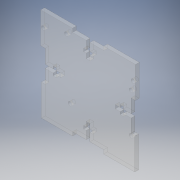
# Autodesk Inventor part: pared lateral
Saved by Autodesk Inventor 2016 (Build 200138000, 138)
## iProperties
Created: 2017-02-20
Part Number: pared lateral
Material: Generic
Document SubType Name: Modeling
Designer: jorge
Density: 1 g/cm^3
Appearance: Clear - Light
Author: jorge
## iProperties of the stored document pared lateral_3DPrint.ipt
Created: 2017-03-11
Part Number: pared lateral_3DPrint
Material: Generic
Document SubType Name: Modeling
Designer: jorge
Density: 1 g/cm^3
Appearance: Default
Author: jorge
Autodesk Inventor part; units mm, degrees
ref_plane "YZ Plane" through (0, 0, 0) normal (1, 0, 0) x (0, 1, 0)
ref_plane "XZ Plane" through (0, 0, 0) normal (0, 1, 0) x (-1, 0, 0)
ref_plane "XY Plane" through (0, 0, 0) normal (0, 0, 1) x (1, 0, 0)
sketch "Sketch1" plane through (0, 0, 0) normal (0, 0, 1) x (1, 0, 0)
  line L0 (0, 0) -> (25, 0) projected
  line L1 (25, 0) -> (25, 3) projected
  line L2 (0, 3) -> (25, 3) projected
  line L3 (0, 0) -> (0, 3) projected
  line L4 (25, 0) -> (50, 0) projected
  line L5 (50, 0) -> (50, 3) projected
  line L6 (25, 3) -> (50, 3) projected
  line L7 (25, 0) -> (25, 3) projected
  line L8 (50, 0) -> (75, 0) projected
  line L9 (75, 0) -> (75, 3) projected
  line L10 (50, 3) -> (75, 3) projected
  line L11 (50, 0) -> (50, 3) projected
  line L12 (0, 0) -> (0, 75)
  line L13 (0, 75) -> (75, 75)
  line L14 (75, 75) -> (75, 0)
  line L15 (75, 0) -> (50, 0)
  line L16 (50, 3) -> (50, 0)
  line L17 (50, 3) -> (25, 3)
  line L18 (25, 3) -> (25, 0)
  line L19 (25, 0) -> (0, 0)
  line L20 (0, 0) -> (0, 25)
  line L21 (0, 25) -> (3, 25)
  line L22 (3, 25) -> (3, 50)
  line L23 (3, 50) -> (0, 50)
  line L24 (25, 75) -> (25, 72)
  line L25 (25, 72) -> (50, 72)
  line L26 (50, 75) -> (50, 72)
  line L27 (75, 50) -> (72, 50)
  line L28 (72, 50) -> (72, 25)
  line L29 (72, 25) -> (75, 25)
  dimension "d0" = 75
  dimension "d1" = 75
  dimension "d2" = 25
  dimension "d3" = 3
  dimension "d4" = 25
  dimension "d5" = 3
  dimension "d6" = 3
  constraints: 36 end point, 11 perpendicular, 6 point on line, 2 collinear, 2 vertical, 1 horizontal
  measures "d0" distance of L0.start L12.end
  measures "d1" distance of L12.end L13.end
  measures "d2" distance of L0.start L20.end
  measures "d3" distance of L20.end L21.end
  measures "d4" distance of L21.end L22.end
  measures "d5" distance of L24.start L24.end
  measures "d6" distance of L27.start L27.end
extrude "Extrusion1" add sketch "Sketch1" along normal blind 3 contours L3 L2 L1 L0 | L12 L21 L22 L23 L13 L24 L25 L26 L14 L27 L28 L29 L10 L6 L2 | L5 L10 L9 L8
sketch "Sketch2" plane through (0, 0, 0) normal (0, 0, -1) x (-1, 0, 0)
  circle A0 centre (-72, 55.2929) radius 1.5 projected
  circle A1 centre (-20, 68.5) radius 1.5 projected
  circle A2 centre (-23, 21.5) radius 1.5 projected
  circle A3 centre (-72, 23.7071) radius 1.5 projected
  point P0 (0, 0)
extrude "Extrusion2" cut sketch "Sketch2" against normal blind 25.4
sketch "Sketch3" plane through (0, 0, 0) normal (0, 0, -1) x (-1, 0, 0)
  line L0 (-50, 72) -> (-39, 72) projected
  line L1 (-25, 72) -> (-25, 75) projected
  line L2 (-25, 75) -> (0, 75) projected
  line L3 (0, 62.5) -> (0, 50) projected
  line L4 (0, 50) -> (-3, 50) projected
  line L5 (-3, 50) -> (-3, 39) projected
  line L6 (-3, 25) -> (0, 25) projected
  line L7 (0, 25) -> (0, 0) projected
  line L8 (0, 0) -> (-25, 0) projected
  line L9 (-25, 0) -> (-25, 3) projected
  line L10 (-25, 3) -> (-36, 3) projected
  line L11 (-50, 3) -> (-50, 0) projected
  line L12 (-50, 0) -> (-75, 0) projected
  line L13 (-75, 0) -> (-75, 25) projected
  line L14 (-75, 25) -> (-72, 25) projected
  line L15 (-72, 25) -> (-72, 36) projected
  line L16 (-72, 50) -> (-75, 50) projected
  line L17 (-75, 62.5) -> (-75, 75) projected
  line L18 (-75, 75) -> (-50, 75) projected
  line L19 (-50, 75) -> (-50, 72) projected
  circle A0 centre (-19, 19.65) radius 1.5 projected
  circle A1 centre (-19, 56.95) radius 1.5 projected
  circle A2 centre (-56.3, 56.95) radius 1.5 projected
  circle A3 centre (-56.3, 19.65) radius 1.5 projected
  line L20 (-39, 72) -> (-36, 72)
  line L21 (-3, 39) -> (-3, 36)
  line L22 (-3, 50) -> (-3, 25) projected
  line L23 (-39, 3) -> (-36, 3)
  line L24 (-25, 3) -> (-50, 3) projected
  line L25 (-72, 36) -> (-72, 39)
  line L26 (-72, 25.2071) -> (-72, 50) projected
  line L27 (-72, 39) -> (-72, 50) projected
  line L28 (-36, 72) -> (-25, 72) projected
  line L29 (-3, 36) -> (-3, 25) projected
  line L30 (-39, 3) -> (-50, 3) projected
  line L31 (-72, 36) -> (-65.65, 36) projected
  line L32 (-65.65, 36) -> (-65.65, 34) projected
  line L33 (-65.65, 34) -> (-63.15, 34) projected
  line L34 (-63.15, 34) -> (-63.15, 36) projected
  line L35 (-63.15, 36) -> (-59.3, 36) projected
  line L36 (-59.3, 36) -> (-59.3, 39) projected
  line L37 (-59.3, 39) -> (-63.15, 39) projected
  line L38 (-63.15, 39) -> (-63.15, 41) projected
  line L39 (-63.15, 41) -> (-65.65, 41) projected
  line L40 (-65.65, 41) -> (-65.65, 39) projected
  line L41 (-65.65, 39) -> (-72, 39) projected
  line L42 (-39, 72) -> (-39, 65.65) projected
  line L43 (-39, 65.65) -> (-41, 65.65) projected
  line L44 (-41, 65.65) -> (-41, 63.15) projected
  line L45 (-41, 63.15) -> (-39, 63.15) projected
  line L46 (-39, 63.15) -> (-39, 59.3) projected
  line L47 (-39, 59.3) -> (-36, 59.3) projected
  line L48 (-36, 59.3) -> (-36, 63.15) projected
  line L49 (-36, 63.15) -> (-34, 63.15) projected
  line L50 (-34, 63.15) -> (-34, 65.65) projected
  line L51 (-34, 65.65) -> (-36, 65.65) projected
  line L52 (-36, 65.65) -> (-36, 72) projected
  line L53 (-3, 39) -> (-9.35, 39) projected
  line L54 (-9.35, 39) -> (-9.35, 41) projected
  line L55 (-9.35, 41) -> (-11.85, 41) projected
  line L56 (-11.85, 41) -> (-11.85, 39) projected
  line L57 (-11.85, 39) -> (-15.7, 39) projected
  line L58 (-15.7, 39) -> (-15.7, 36) projected
  line L59 (-15.7, 36) -> (-11.85, 36) projected
  line L60 (-11.85, 36) -> (-11.85, 34) projected
  line L61 (-11.85, 34) -> (-9.35, 34) projected
  line L62 (-9.35, 34) -> (-9.35, 36) projected
  line L63 (-9.35, 36) -> (-3, 36) projected
  line L64 (-36, 3) -> (-36, 9.35) projected
  line L65 (-36, 9.35) -> (-34, 9.35) projected
  line L66 (-34, 9.35) -> (-34, 11.85) projected
  line L67 (-34, 11.85) -> (-36, 11.85) projected
  line L68 (-36, 11.85) -> (-36, 15.7) projected
  line L69 (-36, 15.7) -> (-39, 15.7) projected
  line L70 (-39, 15.7) -> (-39, 11.85) projected
  line L71 (-39, 11.85) -> (-41, 11.85) projected
  line L72 (-41, 11.85) -> (-41, 9.35) projected
  line L73 (-41, 9.35) -> (-39, 9.35) projected
  line L74 (-39, 9.35) -> (-39, 3) projected
  line L75 (-75, 50) -> (-75, 62.5) projected
  circle A4 centre (-73.5, 62.5) radius 1.5 projected
  line L76 (0, 75) -> (0, 62.5) projected
  circle A5 centre (-1.5, 62.5) radius 1.5 projected
  constraints: 8 end point, 3 collinear
extrude "Extrusion3" cut sketch "Sketch3" against normal blind 25.4 contours L20 L52 L51 L50 L49 L48 L47 L46 L45 L44 L43 L42 | L41 L40 L39 L38 L37 L36 L35 L34 L33 L32 L31 L25 | L21 L63 L62 L61 L60 L59 L58 L57 L56 L55 L54 L53 | L74 L73 L72 L71 L70 L69 L68 L67 L66 L65 L64 L23
sketch "Sketch4" plane through (0, 0, 0) normal (0, 0, -1) x (-1, 0, 0)
  line L0 (-75, 61) -> (-75, 64) projected
  line L1 (0, 65) -> (0, 61.8364) projected
  line L2 (-75, 62.5) -> (-73.5, 62.5)
  line L3 (0, 63.4182) -> (-1.5, 63.4182)
  circle A0 centre (-73.5, 62.5) radius 1.5
  circle A1 centre (-1.5, 63.4182) radius 1.5
  point P0 (0, 0)
  dimension "d13" = 1.5
  dimension "d14" = 1.5
  dimension "d15" = 3
  constraints: 4 end point, 2 coincident, 2 horizontal, 2 midpoint, 1 centre point, 1 horizontal alignment, 2 other
  measures "d13" distance of L2.start L2.end
  measures "d14" distance of L3.start L3.end
  measures "d15" diameter of A0
extrude "Extrusion4" cut sketch "Sketch4" against normal blind 25.4
sketch "Sketch5" plane through (75, 75, 3) normal (1, 0, 0) x (0, 0, -1)
  line L0 (3, -12.5) -> (0, -12.5) projected
  line L1 (3, -12.5) -> (3, 0) projected
  line L2 (3, 0) -> (0, 0) projected
  line L3 (0, -12.5) -> (0, 0) projected
  line L4 (0, -25) -> (0, -12.5) projected
  line L5 (3, -25) -> (0, -25) projected
  line L6 (3, -25) -> (3, -12.5) projected
  point P0 (3, -75)
extrude "Extrusion5" add sketch "Sketch5" along normal blind 0.5
sketch "Sketch6" plane through (0, 75, 0) normal (-1, 0, 0) x (0, 0, 1)
  line L0 (0, -11.5818) -> (3, -11.5818) projected
  line L1 (3, 0) -> (3, -11.5818) projected
  line L2 (0, 0) -> (3, 0) projected
  line L3 (0, 0) -> (0, -11.5818) projected
  line L4 (0, -11.5818) -> (0, -25) projected
  line L5 (0, -25) -> (3, -25) projected
  line L6 (3, -11.5818) -> (3, -25) projected
  point P0 (0, -75)
extrude "Extrusion6" add sketch "Sketch6" along normal blind 0.5
body "Solid1"
